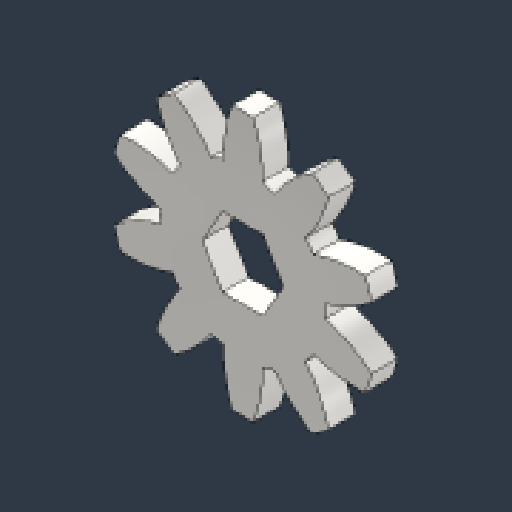
# Autodesk Inventor part: PINION
Saved by Autodesk Inventor 2026 (Build 300175050, 175E)
## iProperties
CustomPartVersion: 1
Created: 2026-04-12
Part Number: PINION
Material: Steel
Document SubType Name: Modeling
Designer: Jthib
Categories: <?xml version="1.0" encoding="UTF-16"?> <MemberInstance><Categories><FamilyTemplate><FamilyTemplateParameter ValueType="xs:double" Id="1" ObjectReferenceKey="da_z" ObjectType="kUserParameterObject"/><FamilyTemplateParameter ValueType="xs:double" Id="2" ObjectReferenceKey="da_b" ObjectType="kUserParameterObject"/><FamilyTemplateParameter ValueType="xs:double" Id="3" ObjectReferenceKey="da_beta" ObjectType="kUserParameterObject"/><FamilyTemplateParameter ValueType="xs:double" Id="4" ObjectReferenceKey="da_da" ObjectType="kUserParameterObject"/><FamilyTemplateParameter ValueType="xs:double" Id="5" ObjectReferenceKey="da_aw" ObjectType="kUserParameterObject"/><FamilyTemplateParameter ValueType="xs:string" Id="6" ObjectReferenceKey="EAIAABAAAAC/AAAAAAAAAIAAAAAAAAAA" ObjectType="83910656" SubObjectId="SurfaceGeometry"/></FamilyTemplate><ParamToTemplateMap><ParamToTemplate CategoryParameter="//CategoryParameter[@InternalName='046C89C9-8512-4d59-83FE-43B91F4F132A']" TemplateParameter="1"/><ParamToTemplate CategoryParameter="//CategoryParameter[@InternalName='2552DF32-E462-4b46-AEBF-C6C7768E72AC']" TemplateParameter="2"/><ParamToTemplate CategoryParameter="//CategoryParameter[@InternalName='C9EE641D-15FC-4fae-A226-E94C4372FDD7']" TemplateParameter="3"/><ParamToTemplate><ParamToTemplate CategoryParameter="//CategoryParameter[@InternalName='00B6519A-459B-49c7-AD84-2E56D39A5744']" ConstantValue="-0.004853"/></ParamToTemplate><ParamToTemplate><ParamToTemplate CategoryParameter="//CategoryParameter[@InternalName='04B31F0E-C7A6-4894-AA32-9629BEFACF47']" ConstantValue="1.000000"/></ParamToTemplate><ParamToTemplate><ParamToTemplate CategoryParameter="//CategoryParameter[@InternalName='43CBEC2E-7847-49e7-A936-2F7889FCB2D9']" ConstantValue="0.250000"/></ParamToTemplate><ParamToTemplate><ParamToTemplate CategoryParameter="//CategoryParameter[@InternalName='B1EFC894-105D-4ebd-86BF-FA20ED196853']" ConstantValue="0.350000"/></ParamToTemplate><ParamToTemplate><ParamToTemplate CategoryParameter="//CategoryParameter[@InternalName='51175063-3D10-4879-93E8-6246FE8B403D']" ConstantValue="2061532430.657340"/></ParamToTemplate><ParamToTemplate><ParamToTemplate CategoryParameter="//CategoryParameter[@InternalName='A3A52E27-4454-46a9-B0BD-C932399B70AF']" ConstantValue="0.300000"/></ParamToTemplate><ParamToTemplate><ParamToTemplate CategoryParameter="//CategoryParameter[@InternalName='91B76062-C214-41d9-B1B9-14D2AB99603D']" ConstantValue="0.400000"/></ParamToTemplate><ParamToTemplate><ParamToTemplate CategoryParameter="//CategoryParameter[@InternalName='374E806E-8B8A-4dda-A9AA-1039D6500AD2']" ConstantValue="2.500000"/></ParamToTemplate><ParamToTemplate><ParamToTemplate CategoryParameter="//CategoryParameter[@InternalName='2D373A89-B862-43d6-8D0B-0CBF12AB9F6C']" ConstantValue="0.349066"/></ParamToTemplate><ParamToTemplate CategoryParameter="//CategoryParameter[@InternalName='37777632-D6A2-4fac-9D53-DB8ACD95C989']" TemplateParameter="4"/><ParamToTemplate CategoryParameter="//CategoryParameter[@InternalName='FD1017F1-B727-4f7e-9707-0F86F1FF9423']" TemplateParameter="5"/><ParamToTemplate><ParamToTemplate CategoryParameter="//CategoryParameter[@InternalName='9E1B4470-B2D3-4ff1-B813-535BB4CDF51A']" ConstantValue="3523220.976809"/></ParamToTemplate><ParamToTemplate><ParamToTemplate CategoryParameter="//CategoryParameter[@InternalName='F8452263-BFF6-458c-9FB1-07C4B99E95CD']" ConstantValue="11397033.805607"/></ParamToTemplate><ParamToTemplate><ParamToTemplate CategoryParameter="//CategoryParameter[@InternalName='3E3BB259-FD49-497f-8171-6EBC954A3479']" ConstantValue="2.000000"/></ParamToTemplate><ParamToTemplate CategoryParameter="//CategoryParameter[@InternalName='27C3BAF2-7550-4e4b-AE2C-0DB134B7D9B7']" TemplateParameter="6"/></ParamToTemplateMap><Category DisplayName="Gear" InternalName="DC85795E-93AB-48d5-8EEE-5A27447B64BD" Mnemonic="Gear"><CategoryParameter DisplayName="z" InternalName="046C89C9-8512-4d59-83FE-43B91F4F132A" Mnemonic="z"/><CategoryParameter DisplayName="b" InternalName="2552DF32-E462-4b46-AEBF-C6C7768E72AC" Mnemonic="b"/><CategoryParameter DisplayName="||b|" InternalName="C9EE641D-15FC-4fae-A226-E94C4372FDD7" Mnemonic="beta"/><CategoryParameter DisplayName="x" InternalName="00B6519A-459B-49c7-AD84-2E56D39A5744" Mnemonic="x"/><CategoryParameter DisplayName="a*" InternalName="04B31F0E-C7A6-4894-AA32-9629BEFACF47" Mnemonic="a"/><CategoryParameter DisplayName="c*" InternalName="43CBEC2E-7847-49e7-A936-2F7889FCB2D9" Mnemonic="c"/><CategoryParameter DisplayName="r|.f|*" InternalName="B1EFC894-105D-4ebd-86BF-FA20ED196853" Mnemonic="rf"/><CategoryParameter DisplayName="E" InternalName="51175063-3D10-4879-93E8-6246FE8B403D" Mnemonic="E"/><CategoryParameter DisplayName="||m|" InternalName="A3A52E27-4454-46a9-B0BD-C932399B70AF" Mnemonic="mi"/><Category DisplayName="SpurGear" InternalName="26C5A22E-A91E-4dfd-A3B3-23CCAFAE1764" Mnemonic="SpurGear"><CategoryParameter DisplayName="m" InternalName="91B76062-C214-41d9-B1B9-14D2AB99603D" Mnemonic="m"/><CategoryParameter DisplayName="P" InternalName="374E806E-8B8A-4dda-A9AA-1039D6500AD2" Mnemonic="PP"/><CategoryParameter DisplayName="||a|" InternalName="2D373A89-B862-43d6-8D0B-0CBF12AB9F6C" Mnemonic="alpha"/><CategoryParameter DisplayName="d|.a|" InternalName="37777632-D6A2-4fac-9D53-DB8ACD95C989" Mnemonic="da"/><CategoryParameter DisplayName="a|.w|" InternalName="FD1017F1-B727-4f7e-9707-0F86F1FF9423" Mnemonic="aw"/><CategoryParameter DisplayName="||s||.Flim|" InternalName="9E1B4470-B2D3-4ff1-B813-535BB4CDF51A" Mnemonic="sFlim"/><CategoryParameter DisplayName="||s||.Hlim|" InternalName="F8452263-BFF6-458c-9FB1-07C4B99E95CD" Mnemonic="sHlim"/><CategoryParameter DisplayName="type" InternalName="3E3BB259-FD49-497f-8171-6EBC954A3479" Mnemonic="type"/><CategoryParameter DisplayName="PitchDiameter" InternalName="27C3BAF2-7550-4e4b-AE2C-0DB134B7D9B7" Mnemonic="IDS_PITCHDIAM"/></Category></Category></Categories></MemberInstance>
Mass: 39.5051 g
Surface Area: 34.6827 cm^2
Volume: 5.0325 cm^3
Density: 7.85 g/cm^3
Appearance: Steel
Author: Jthib
Autodesk Inventor part; units mm, degrees
sketch "Sketch1" plane through (0, 0, 0) normal (0, 0, 1) x (1, 0, 0)
  circle A0 centre (0, 0) radius 23.8125
  dimension "d0" = 47.625
  constraints: 1 centre point
  measures "d0" diameter of A0
extrude "Extrusion1" add sketch "Sketch1" along normal blind 4.7625
sketch "Sketch2" plane through (0, 0, 0) normal (0, 0, -1) x (-1, 0, 0)
  circle A0 centre (0, 0) radius 23.8125 projected
  circle A1 centre (0, 0) radius 20
  dimension "d3" = 40
  constraints: 1 centre point, 1 coincident
  measures "d3" diameter of A1
surface extrude "Pitch Diameter" sketch "Sketch2" against normal through all shown no curves A1
ref_plane "Work Plane1" through (0, 0, 0) normal (1, 0, 0) x (0, 1, 0)
ref_plane "Work Plane2" through (0, 0, 0) normal (0.9510565, 0.309017, 0) x (0, 0, 1)
ref_plane "Work Plane3" through (0, 0, 2.3813) normal (0, 0, -1) x (-1, 0, 0)
feature "Spur Gear" [suppressed]
sketch "Sketch3" plane through (0, 0, 4.7625) normal (0, 0, 1) x (1, 0, 0)
  line L0 (-7.3323, 0) -> (-3.6662, 6.35)
  line L1 (-3.6662, 6.35) -> (3.6662, 6.35)
  line L2 (3.6662, 6.35) -> (7.3323, 0)
  line L3 (7.3323, 0) -> (3.6662, -6.35)
  line L4 (3.6662, -6.35) -> (-3.6662, -6.35)
  line L5 (-3.6662, -6.35) -> (-7.3323, 0)
  point P0 (0, 0)
  point P1 (0, 0)
  dimension "d20" = 12.7
  constraints: 12 end point, 1 coincident, 1 horizontal alignment, 13 other
  measures "d20" distance between parallel lines of L3 L0
extrude "Extrusion2" cut sketch "Sketch3" along normal through all both and the other way through all
sketch "Sketch4" plane through (0, 0, 4.7625) normal (0, 0, 1) x (1, 0, 0)
  spline S0 degree 3 poles (-6.2781, 23.1442) (-6.0859, 22.9986) (-5.7015, 22.7075) (-5.155, 22.2331) (-4.6341, 21.7312) (-4.1451, 21.1978) (-3.6931, 20.6326) (-3.3541, 20.1335) (-3.1114, 19.7167) (-2.9473, 19.3945) (-2.8005, 19.0634) (-2.73, 18.8328) (-2.6947, 18.7174) knots 0 0 0 0 0.072314 0.144628 0.216942 0.289253 0.36156 0.433862 0.47002 0.506176 0.54233 0.578472 0.578472 0.578472 0.578472
  spline S1 degree 3 poles (-2.6947, 18.7174) (-2.7004, 18.4978) (-2.7088, 18.1683) (-2.6724, 17.7302) (-2.6224, 17.4046) (-2.5569, 17.0815) (-2.4597, 16.7664) (-2.3407, 16.459) (-2.1912, 16.1648) (-2.0093, 15.8895) (-1.7965, 15.6372) (-1.5519, 15.4152) (-1.276, 15.2336) (-0.9768, 15.0933) (-0.7109, 15.0216) (-0.4942, 14.9855) (-0.2744, 14.9772) (0, 14.9828) (0.2744, 14.9772) (0.4942, 14.9855) (0.7109, 15.0216) (0.9768, 15.0933) (1.276, 15.2336) (1.5519, 15.4152) (1.7965, 15.6372) (2.0093, 15.8895) (2.1912, 16.1648) (2.3407, 16.459) (2.4597, 16.7664) (2.5569, 17.0815) (2.6224, 17.4046) (2.6724, 17.7302) (2.7088, 18.1683) (2.7004, 18.4978) (2.6947, 18.7174) knots 0 0 0 0 0.065852 0.098787 0.13172 0.164652 0.197584 0.230508 0.263442 0.296373 0.329294 0.362209 0.395115 0.428021 0.460912 0.477386 0.49385 0.526785 0.55972 0.576184 0.592658 0.625549 0.658455 0.691362 0.724276 0.757197 0.790128 0.823062 0.855987 0.888918 0.92185 0.954783 0.987718 1.05357 1.05357 1.05357 1.05357
  spline S2 degree 3 poles (2.6947, 18.7174) (2.73, 18.8328) (2.8005, 19.0634) (2.9473, 19.3945) (3.1114, 19.7167) (3.3541, 20.1335) (3.6931, 20.6326) (4.1451, 21.1978) (4.6341, 21.7312) (5.155, 22.2331) (5.7015, 22.7075) (6.0859, 22.9986) (6.2781, 23.1442) knots 0 0 0 0 0.036142 0.072296 0.108452 0.14461 0.216912 0.28922 0.361531 0.433844 0.506158 0.578472 0.578472 0.578472 0.578472
  circle A0 centre (0, 0) radius 14.9806 construction
  circle A1 centre (0, 0) radius 18.7939 construction
  circle A2 centre (0, 0) radius 20 construction
  circle A3 centre (0, 0) radius 23.9806
  point P0 (-5.7065, 22.7013)
  point P1 (-5.1593, 22.2285)
  point P2 (-4.6394, 21.7259)
  point P3 (-4.1512, 21.1924)
  point P4 (-3.7006, 20.6269)
  point P5 (-3.2958, 20.0279)
  point P6 (-3.1144, 19.7151)
  point P7 (-2.9502, 19.393)
  point P8 (-2.8073, 19.0609)
  point P9 (-2.6957, 18.0589)
  point P10 (-2.6686, 17.7307)
  point P11 (-2.6198, 17.405)
  point P12 (-2.5516, 17.0828)
  point P13 (-2.456, 16.7677)
  point P14 (-2.3356, 16.4612)
  point P15 (-2.1858, 16.168)
  point P16 (-2.0041, 15.8933)
  point P17 (-1.7912, 15.6422)
  point P18 (-1.5467, 15.4219)
  point P19 (-1.2721, 15.2405)
  point P20 (-0.9735, 15.1023)
  point P21 (-0.6565, 15.0144)
  point P22 (-0.4938, 14.989)
  point P23 (-0.3294, 14.9803)
  point P24 (0, 14.9806)
  point P25 (0.3294, 14.9803)
  point P26 (0.4938, 14.989)
  point P27 (0.6565, 15.0144)
  point P28 (0.9735, 15.1023)
  point P29 (1.2721, 15.2405)
  point P30 (1.5467, 15.4219)
  point P31 (1.7912, 15.6422)
  point P32 (2.0041, 15.8933)
  point P33 (2.1858, 16.168)
  point P34 (2.3356, 16.4612)
  point P35 (2.456, 16.7677)
  point P36 (2.5516, 17.0828)
  point P37 (2.6198, 17.405)
  point P38 (2.6686, 17.7307)
  point P39 (2.6957, 18.0589)
  point P40 (2.8073, 19.0609)
  point P41 (2.9502, 19.393)
  point P42 (3.1144, 19.7151)
  point P43 (3.2958, 20.0279)
  point P44 (3.7006, 20.6269)
  point P45 (4.1512, 21.1924)
  point P46 (4.6394, 21.7259)
  point P47 (5.1593, 22.2285)
  point P48 (5.7065, 22.7013)
  constraints: 4 centre point, 2 point on circle, 113 other
extrude "Extrusion3" cut sketch "Sketch4" against normal through all contours A3 S2 S1 S0 picked at (0.7325, 21.0862)
pattern_circular "Circular Pattern1" count 10 over 360 about axis through (0, 0, 0) along (0, 0, 1) of "Extrusion3"
fillet "Fillet2" radius 1.5875 4 edges at (-8.5862, 22.2106, 2.3812) (-6.1087, 23.0156, 2.3813) (-2.6947, 18.7174, 2.3813) (-8.8218, 16.7266, 2.3812)
pattern_circular "Circular Pattern3" count 10 over 360 about axis through (0, 0, 0) along (0, 0, 1) of "Fillet2"
sketch "Sketch5" plane through (0, 0, 0) normal (0, 0, 1) x (1, 0, 0)
  circle A0 centre (0, 0) radius 20 construction
  dimension "d36" = 40
  constraints: 1 centre point, 1 coincident
  measures "d36" diameter of A0
equation "\"d0\" = da_da"
equation "\"d1\" = da_b"
equation "\"d36\" = da_d"
equation "\"d3\" = da_d"
equation "\"d15\" = da_aw"
equation "\"d19\" = da_aw"
equation "\"da_da\" = 47.625"
equation "\"da_b\" = 4.7625"
equation "\"da_d\" = 40"
equation "\"da_aw\" = 746.76"
body "Solid1"
body "Srf1"
